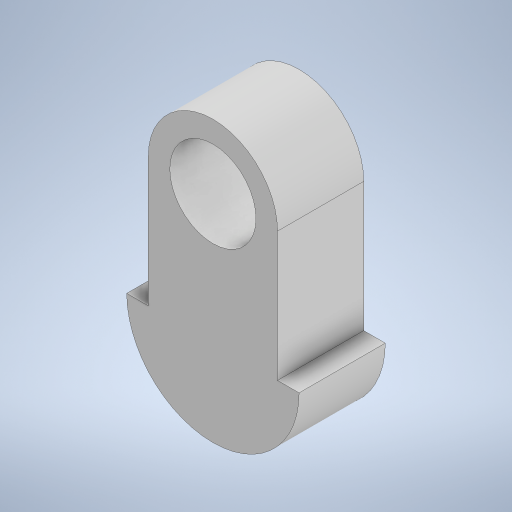
# Autodesk Inventor part: khurramf_01_Swing
Saved by Autodesk Inventor 2024 (Build 280153000, 153)
## iProperties
Created: 2024-01-30
Part Number: khurramf_01_Swing
Material: Generic
Document SubType Name: Modeling
Designer: furqa
Density: 1 g/cm^3
Appearance: Default
Author: furqa
Autodesk Inventor part; units mm, degrees
ref_plane "YZ Plane" through (0, 0, 0) normal (1, 0, 0) x (0, 1, 0)
ref_plane "XZ Plane" through (0, 0, 0) normal (0, 1, 0) x (-1, 0, 0)
ref_plane "XY Plane" through (0, 0, 0) normal (0, 0, 1) x (1, 0, 0)
sketch "Sketch1" plane through (0, 0, 0) normal (0, 0, 1) x (1, 0, 0)
  line L0 (-6, 0) -> (-6, 12)
  line L1 (-8, 0) -> (-6, 0)
  line L2 (8, 0) -> (6, 0)
  line L3 (6, 0) -> (6, 12)
  arc A0 (-8, 0) -> (8, 0) centre (0, 0) ccw
  arc A1 (6, 12) -> (-6, 12) centre (0, 12) ccw
  circle A2 centre (0, 12) radius 4
  point P0 (0, -8)
  dimension "d1" = 2
  dimension "d2" = 8
  dimension "d3" = 2
  dimension "d9" = 20
  constraints: 8 end point, 5 point on circle, 3 centre point, 2 coincident, 2 point on line, 1 horizontal, 1 perpendicular, 1 vertical
  measures "d1" distance of L1.start L0.start
  measures "d2" radius of A0
  measures "d3" distance of L2.start L2.end
  measures "d9" distance of point (0, -8) A1.centre
extrude "Extrusion1" add sketch "Sketch1" along normal blind 8
body "Solid1"
